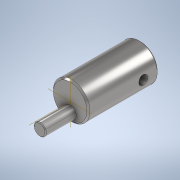
# Autodesk Inventor part: crankshaft valve crank
Saved by Autodesk Inventor 2021.1 (Build 251245000, 245)
## iProperties
Created: 2020-08-31
Part Number: crankshaft valve crank
Material: Stainless Steel
Document SubType Name: Sheet Metal
Designer: Vamshi
Mass: 345.211 g
Surface Area: 83.3047 cm^2
Volume: 43.1513 cm^3
Density: 8 g/cm^3
Sheet Metal Rule: Default
Appearance: Semi-Polished
Author: Vamshi
Autodesk Inventor part; units mm, degrees
ref_plane "YZ Plane" through (0, 0, 0) normal (1, 0, 0) x (0, 1, 0)
ref_plane "XZ Plane" through (0, 0, 0) normal (0, 1, 0) x (-1, 0, 0)
ref_plane "XY Plane" through (0, 0, 0) normal (0, 0, 1) x (1, 0, 0)
sketch "Sketch1" plane through (0, 0, 0) normal (0, 0, 1) x (1, 0, 0)
  circle A0 centre (0, 0) radius 15.24
  circle A1 centre (0, -7.62) radius 5.08
  dimension "d0" = 30.48
  dimension "d1" = 10.16
  dimension "d2" = 7.62
  constraints: 2 centre point, 1 coincident
  measures "d0" diameter of A0
  measures "d1" diameter of A1
  measures "d2" distance of A1.centre point (0, 0)
extrude "Extrusion1" add sketch "Sketch1" against normal blind 58.42 contours A0 | A1
extrude "Extrusion2" add sketch "Sketch1" along normal blind 25.4 contours A1
sketch "Sketch2" plane through (0, 0, 0) normal (1, 0, 0) x (0, 1, 0)
  line L0 (15.24, 0) -> (15.24, -58.42) projected
  line L1 (15.24, -58.42) -> (-15.24, -58.42) projected
  line L2 (-15.24, -58.42) -> (-15.24, 0) projected
  line L3 (-15.24, 0) -> (-12.7, 0) projected
  line L4 (-12.7, 0) -> (-12.7, 25.4) projected
  line L5 (-12.7, 25.4) -> (-2.54, 25.4) projected
  line L6 (-2.54, 25.4) -> (-2.54, 0) projected
  line L7 (-2.54, 0) -> (15.24, 0) projected
  line L8 (-15.24, -58.42) -> (15.24, -58.42) projected
  line L9 (15.24, 0) -> (-15.24, 0) projected
  circle A0 centre (0, -45.72) radius 3.81
  point P0 (0, 0)
  dimension "d7" = 7.62
  dimension "d8" = 12.7
  constraints: 1 centre point
  measures "d7" diameter of A0
  measures "d8" distance from line of A0.centre L1
extrude "Extrusion3" cut sketch "Sketch2" against normal through all both and the other way through all contours A0
chamfer "Chamfer1" distance 0.635 angle 45 1 edges at (-5.08, -7.62, 25.4) measured on face at (5.0635, -8.0288, 16.9333)
chamfer "Chamfer2" distance 1.27 angle 45 2 edges at (-15.24, 0, -58.42) (-15.24, 0, 0) measured on face at (9.6385, 11.805, -38.9467)
equation "\"BendRadius\" = Thickness"
equation "\"BendReliefWidth\" = Thickness"
equation "\"BendReliefDepth\" = 0.5 * Thickness"
equation "\"CornerReliefSize\" = 4 * Thickness"
equation "\"MinimumRemnant\" = 2 * Thickness"
equation "\"TransitionRadius\" = BendRadius"
equation "\"JacobiRadiusSize\" = BendRadius"
equation "\"GapSize\" = Thickness"
equation "\"Thickness\" = 3.048"
body "Solid1"
